Autodesk Fusion 360 part; units mm, degrees
(part 13 of 40)
  line L5726 (150.1623, 135.5673) -> (150.0253, 135.4891) construction
  line L5727 (150.0253, 135.4891) -> (149.8888, 135.4096) construction
  line L5728 (149.8888, 135.4096) -> (149.7528, 135.3289) construction
  line L5729 (149.7528, 135.3289) -> (149.6172, 135.247) construction
  line L5730 (149.6172, 135.247) -> (149.4822, 135.1637) construction
  line L5731 (149.4822, 135.1637) -> (149.3477, 135.0792) construction
  line L5732 (149.3477, 135.0792) -> (149.2136, 134.9936) construction
  line L5733 (149.2136, 134.9936) -> (149.08, 134.9068) construction
  line L5734 (149.08, 134.9068) -> (148.9468, 134.819) construction
  line L5735 (148.9468, 134.819) -> (148.814, 134.7302) construction
  line L5736 (148.814, 134.7302) -> (148.6817, 134.6403) construction
  line L5737 (148.6817, 134.6403) -> (148.5499, 134.5494) construction
  line L5738 (148.5499, 134.5494) -> (148.4185, 134.4575) construction
  line L5739 (148.4185, 134.4575) -> (148.2875, 134.3646) construction
  line L5740 (148.2875, 134.3646) -> (148.157, 134.2707) construction
  line L5741 (148.157, 134.2707) -> (148.027, 134.1758) construction
  line L5742 (148.027, 134.1758) -> (147.8974, 134.08) construction
  line L5743 (147.8974, 134.08) -> (147.7682, 133.9832) construction
  line L5744 (147.7682, 133.9832) -> (147.6394, 133.8854) construction
  line L5745 (147.6394, 133.8854) -> (147.5111, 133.7868) construction
  line L5746 (147.5111, 133.7868) -> (147.3832, 133.6873) construction
  line L5747 (147.3832, 133.6873) -> (147.2558, 133.5869) construction
  line L5748 (147.2558, 133.5869) -> (147.1288, 133.4856) construction
  line L5749 (147.1288, 133.4856) -> (147.0022, 133.3834) construction
  line L5750 (147.0022, 133.3834) -> (146.876, 133.2804) construction
  line L5751 (146.876, 133.2804) -> (146.7503, 133.1765) construction
  line L5752 (146.7503, 133.1765) -> (146.625, 133.0717) construction
  line L5753 (146.625, 133.0717) -> (146.5002, 132.9662) construction
  line L5754 (146.5002, 132.9662) -> (146.3758, 132.8598) construction
  line L5755 (146.3758, 132.8598) -> (146.2518, 132.7526) construction
  line L5756 (146.2518, 132.7526) -> (146.1282, 132.6445) construction
  line L5757 (146.1282, 132.6445) -> (146.0051, 132.5357) construction
  line L5758 (146.0051, 132.5357) -> (145.8823, 132.4261) construction
  line L5759 (145.8823, 132.4261) -> (145.7601, 132.3158) construction
  line L5760 (145.7601, 132.3158) -> (145.6382, 132.2046) construction
  line L5761 (145.6382, 132.2046) -> (145.5168, 132.0927) construction
  line L5762 (145.5168, 132.0927) -> (145.3958, 131.98) construction
  line L5763 (145.3958, 131.98) -> (145.2752, 131.8665) construction
  line L5764 (145.2752, 131.8665) -> (145.1551, 131.7523) construction
  line L5765 (145.1551, 131.7523) -> (145.0354, 131.6374) construction
  line L5766 (145.0354, 131.6374) -> (144.9161, 131.5218) construction
  line L5767 (144.9161, 131.5218) -> (144.7973, 131.4054) construction
  line L5768 (144.7973, 131.4054) -> (144.6789, 131.2882) construction
  line L5769 (144.6789, 131.2882) -> (144.5609, 131.1704) construction
  line L5770 (144.5609, 131.1704) -> (144.4433, 131.0519) construction
  line L5771 (144.4433, 131.0519) -> (144.3262, 130.9326) construction
  line L5772 (144.3262, 130.9326) -> (144.2095, 130.8127) construction
  line L5773 (144.2095, 130.8127) -> (144.0932, 130.6921) construction
  line L5774 (144.0932, 130.6921) -> (143.9774, 130.5707) construction
  line L5775 (143.9774, 130.5707) -> (143.862, 130.4488) construction
  line L5776 (143.862, 130.4488) -> (143.747, 130.3261) construction
  line L5777 (143.747, 130.3261) -> (143.6553, 130.2274) construction
  line L5778 (143.6553, 130.2274) -> (143.5868, 130.1531) construction
  line L5779 (143.5868, 130.1531) -> (143.5412, 130.1034) construction
  line L5780 (143.5412, 130.1034) -> (143.5184, 130.0785) construction
  arc A153 (161.0254, 119.7202) -> (161.7599, 122.4018) centre (160.0059, 121.4408) ccw
  arc A154 (152.9878, 155.5428) -> (155.1583, 157.2806) centre (153.1745, 157.5341) ccw
  arc A155 (143.5184, 130.0785) -> (144.9129, 125.7868) centre (212.132, 150) ccw
  arc A156 (160.1966, 125.4699) -> (161.7599, 122.4018) centre (212.132, 150) ccw
  line L5781 (152.9878, 155.5428) -> (151.3635, 155.6951)
  arc A157 (154.1697, 136.995) -> (155.697, 139.3184) centre (153.7319, 138.9465) ccw
  arc A158 (155.1583, 142.7194) -> (155.697, 139.3184) centre (212.132, 150) ccw
  spline S77 degree 5 poles (151.3635, 144.3049) (151.3327, 144.3021) (151.2711, 144.2971) (151.1787, 144.2922) (151.0554, 144.2903) (150.901, 144.2944) (150.7464, 144.3031) (150.5917, 144.3146) (150.437, 144.3277) (150.2822, 144.3417) (150.1275, 144.3569) (149.9727, 144.3735) (149.818, 144.392) (149.6632, 144.4129) (149.5085, 144.4359) (149.3538, 144.461) (149.1991, 144.4879) (149.0445, 144.5162) (148.8899, 144.5458) (148.7354, 144.5767) (148.5809, 144.6087) (148.4265, 144.6421) (148.2722, 144.6768) (148.118, 144.7129) (147.9638, 144.7503) (147.8098, 144.7891) (147.6558, 144.8291) (147.5019, 144.8703) (147.3481, 144.9127) (147.1944, 144.9561) (147.0408, 145.0007) (146.8873, 145.0464) (146.734, 145.0932) (146.5807, 145.1411) (146.4276, 145.1901) (146.2746, 145.2401) (146.1217, 145.2913) (145.9689, 145.3434) (145.8162, 145.3965) (145.6637, 145.4507) (145.5114, 145.5058) (145.3591, 145.562) (145.207, 145.619) (145.055, 145.6771) (144.9032, 145.7361) (144.7516, 145.7961) (144.6, 145.857) (144.4487, 145.9188) (144.2975, 145.9815) (144.1464, 146.0452) (143.9955, 146.1097) (143.8448, 146.1751) (143.6942, 146.2415) (143.5438, 146.3087) (143.3936, 146.3767) (143.2435, 146.4457) (143.0936, 146.5154) (142.9439, 146.5861) (142.7944, 146.6575) (142.645, 146.7299) (142.4958, 146.803) (142.3468, 146.877) (142.198, 146.9518) (142.0494, 147.0274) (141.9009, 147.1038) (141.7527, 147.181) (141.6046, 147.259) (141.4568, 147.3378) (141.3091, 147.4174) (141.1617, 147.4977) (141.0144, 147.5789) (140.8968, 147.6444) (140.8086, 147.6939) (140.7499, 147.7271) (140.7205, 147.7437) knots 0 0 0 0 0 0 0.01428571 0.02857143 0.04285714 0.05714286 0.07142857 0.08571429 0.1 0.11428571 0.12857143 0.14285714 0.15714286 0.17142857 0.18571429 0.2 0.21428571 0.22857143 0.24285714 0.25714286 0.27142857 0.28571429 0.3 0.31428571 0.32857143 0.34285714 0.35714286 0.37142857 0.38571429 0.4 0.41428571 0.42857143 0.44285714 0.45714286 0.47142857 0.48571429 0.5 0.51428571 0.52857143 0.54285714 0.55714286 0.57142857 0.58571429 0.6 0.61428571 0.62857143 0.64285714 0.65714286 0.67142857 0.68571429 0.7 0.71428571 0.72857143 0.74285714 0.75714286 0.77142857 0.78571429 0.8 0.81428571 0.82857143 0.84285714 0.85714286 0.87142857 0.88571429 0.9 0.91428571 0.92857143 0.94285714 0.95714286 0.97142857 0.98571429 1 1 1 1 1 1
  line L5782 (151.3635, 144.3049) -> (151.3327, 144.3021) construction
  line L5783 (151.3327, 144.3021) -> (151.2711, 144.2971) construction
  line L5784 (151.2711, 144.2971) -> (151.1787, 144.2922) construction
  line L5785 (151.1787, 144.2922) -> (151.0554, 144.2903) construction
  line L5786 (151.0554, 144.2903) -> (150.901, 144.2944) construction
  line L5787 (150.901, 144.2944) -> (150.7464, 144.3031) construction
  line L5788 (150.7464, 144.3031) -> (150.5917, 144.3146) construction
  line L5789 (150.5917, 144.3146) -> (150.437, 144.3277) construction
  line L5790 (150.437, 144.3277) -> (150.2822, 144.3417) construction
  line L5791 (150.2822, 144.3417) -> (150.1275, 144.3569) construction
  line L5792 (150.1275, 144.3569) -> (149.9727, 144.3735) construction
  line L5793 (149.9727, 144.3735) -> (149.818, 144.392) construction
  line L5794 (149.818, 144.392) -> (149.6632, 144.4129) construction
  line L5795 (149.6632, 144.4129) -> (149.5085, 144.4359) construction
  line L5796 (149.5085, 144.4359) -> (149.3538, 144.461) construction
  line L5797 (149.3538, 144.461) -> (149.1991, 144.4879) construction
  line L5798 (149.1991, 144.4879) -> (149.0445, 144.5162) construction
  line L5799 (149.0445, 144.5162) -> (148.8899, 144.5458) construction
  line L5800 (148.8899, 144.5458) -> (148.7354, 144.5767) construction
  line L5801 (148.7354, 144.5767) -> (148.5809, 144.6087) construction
  line L5802 (148.5809, 144.6087) -> (148.4265, 144.6421) construction
  line L5803 (148.4265, 144.6421) -> (148.2722, 144.6768) construction
  line L5804 (148.2722, 144.6768) -> (148.118, 144.7129) construction
  line L5805 (148.118, 144.7129) -> (147.9638, 144.7503) construction
  line L5806 (147.9638, 144.7503) -> (147.8098, 144.7891) construction
  line L5807 (147.8098, 144.7891) -> (147.6558, 144.8291) construction
  line L5808 (147.6558, 144.8291) -> (147.5019, 144.8703) construction
  line L5809 (147.5019, 144.8703) -> (147.3481, 144.9127) construction
  line L5810 (147.3481, 144.9127) -> (147.1944, 144.9561) construction
  line L5811 (147.1944, 144.9561) -> (147.0408, 145.0007) construction
  line L5812 (147.0408, 145.0007) -> (146.8873, 145.0464) construction
  line L5813 (146.8873, 145.0464) -> (146.734, 145.0932) construction
  line L5814 (146.734, 145.0932) -> (146.5807, 145.1411) construction
  line L5815 (146.5807, 145.1411) -> (146.4276, 145.1901) construction
  line L5816 (146.4276, 145.1901) -> (146.2746, 145.2401) construction
  line L5817 (146.2746, 145.2401) -> (146.1217, 145.2913) construction
  line L5818 (146.1217, 145.2913) -> (145.9689, 145.3434) construction
  line L5819 (145.9689, 145.3434) -> (145.8162, 145.3965) construction
  line L5820 (145.8162, 145.3965) -> (145.6637, 145.4507) construction
  line L5821 (145.6637, 145.4507) -> (145.5114, 145.5058) construction
  line L5822 (145.5114, 145.5058) -> (145.3591, 145.562) construction
  line L5823 (145.3591, 145.562) -> (145.207, 145.619) construction
  line L5824 (145.207, 145.619) -> (145.055, 145.6771) construction
  line L5825 (145.055, 145.6771) -> (144.9032, 145.7361) construction
  line L5826 (144.9032, 145.7361) -> (144.7516, 145.7961) construction
  line L5827 (144.7516, 145.7961) -> (144.6, 145.857) construction
  line L5828 (144.6, 145.857) -> (144.4487, 145.9188) construction
  line L5829 (144.4487, 145.9188) -> (144.2975, 145.9815) construction
  line L5830 (144.2975, 145.9815) -> (144.1464, 146.0452) construction
  line L5831 (144.1464, 146.0452) -> (143.9955, 146.1097) construction
  line L5832 (143.9955, 146.1097) -> (143.8448, 146.1751) construction
  line L5833 (143.8448, 146.1751) -> (143.6942, 146.2415) construction
  line L5834 (143.6942, 146.2415) -> (143.5438, 146.3087) construction
  line L5835 (143.5438, 146.3087) -> (143.3936, 146.3767) construction
  line L5836 (143.3936, 146.3767) -> (143.2435, 146.4457) construction
  line L5837 (143.2435, 146.4457) -> (143.0936, 146.5154) construction
  line L5838 (143.0936, 146.5154) -> (142.9439, 146.5861) construction
  line L5839 (142.9439, 146.5861) -> (142.7944, 146.6575) construction
  line L5840 (142.7944, 146.6575) -> (142.645, 146.7299) construction
  line L5841 (142.645, 146.7299) -> (142.4958, 146.803) construction
  line L5842 (142.4958, 146.803) -> (142.3468, 146.877) construction
  line L5843 (142.3468, 146.877) -> (142.198, 146.9518) construction
  line L5844 (142.198, 146.9518) -> (142.0494, 147.0274) construction
  line L5845 (142.0494, 147.0274) -> (141.9009, 147.1038) construction
  line L5846 (141.9009, 147.1038) -> (141.7527, 147.181) construction
  line L5847 (141.7527, 147.181) -> (141.6046, 147.259) construction
  line L5848 (141.6046, 147.259) -> (141.4568, 147.3378) construction
  line L5849 (141.4568, 147.3378) -> (141.3091, 147.4174) construction
  line L5850 (141.3091, 147.4174) -> (141.1617, 147.4977) construction
  line L5851 (141.1617, 147.4977) -> (141.0144, 147.5789) construction
  line L5852 (141.0144, 147.5789) -> (140.8968, 147.6444) construction
  line L5853 (140.8968, 147.6444) -> (140.8086, 147.6939) construction
  line L5854 (140.8086, 147.6939) -> (140.7499, 147.7271) construction
  line L5855 (140.7499, 147.7271) -> (140.7205, 147.7437) construction
  arc A159 (155.697, 160.6816) -> (154.1697, 163.005) centre (153.7319, 161.0535) ccw
  arc A160 (154.1697, 136.995) -> (155.697, 139.3184) centre (153.7319, 138.9465) ccw
  arc A161 (255.932, 206.4469) -> (252.2812, 209.0993) centre (212.132, 150) ccw
  spline S78 degree 5 poles (152.5778, 163.3622) (152.5477, 163.369) (152.4876, 163.3833) (152.3982, 163.4071) (152.2803, 163.4435) (152.1347, 163.4951) (151.9904, 163.5511) (151.8468, 163.6099) (151.7037, 163.6701) (151.5609, 163.7313) (151.4184, 163.7935) (151.2763, 163.8571) (151.1349, 163.9226) (150.9941, 163.9902) (150.8541, 164.06) (150.7147, 164.1316) (150.5759, 164.205) (150.4376, 164.2797) (150.2998, 164.3557) (150.1623, 164.4327) (150.0253, 164.5109) (149.8888, 164.5904) (149.7528, 164.6711) (149.6172, 164.753) (149.4822, 164.8363) (149.3477, 164.9208) (149.2136, 165.0064) (149.08, 165.0932) (148.9468, 165.181) (148.814, 165.2698) (148.6817, 165.3597) (148.5499, 165.4506) (148.4185, 165.5425) (148.2875, 165.6354) (148.157, 165.7293) (148.027, 165.8242) (147.8974, 165.92) (147.7682, 166.0168) (147.6394, 166.1146) (147.5111, 166.2132) (147.3832, 166.3127) (147.2558, 166.4131) (147.1288, 166.5144) (147.0022, 166.6166) (146.876, 166.7196) (146.7503, 166.8235) (146.625, 166.9283) (146.5002, 167.0338) (146.3758, 167.1402) (146.2518, 167.2474) (146.1282, 167.3555) (146.0051, 167.4643) (145.8823, 167.5739) (145.7601, 167.6842) (145.6382, 167.7954) (145.5168, 167.9073) (145.3958, 168.02) (145.2752, 168.1335) (145.1551, 168.2477) (145.0354, 168.3626) (144.9161, 168.4782) (144.7973, 168.5946) (144.6789, 168.7118) (144.5609, 168.8296) (144.4433, 168.9481) (144.3262, 169.0674) (144.2095, 169.1873) (144.0932, 169.3079) (143.9774, 169.4293) (143.862, 169.5512) (143.747, 169.6739) (143.6553, 169.7726) (143.5868, 169.8469) (143.5412, 169.8966) (143.5184, 169.9215) knots 0 0 0 0 0 0 0.01428571 0.02857143 0.04285714 0.05714286 0.07142857 0.08571429 0.1 0.11428571 0.12857143 0.14285714 0.15714286 0.17142857 0.18571429 0.2 0.21428571 0.22857143 0.24285714 0.25714286 0.27142857 0.28571429 0.3 0.31428571 0.32857143 0.34285714 0.35714286 0.37142857 0.38571429 0.4 0.41428571 0.42857143 0.44285714 0.45714286 0.47142857 0.48571429 0.5 0.51428571 0.52857143 0.54285714 0.55714286 0.57142857 0.58571429 0.6 0.61428571 0.62857143 0.64285714 0.65714286 0.67142857 0.68571429 0.7 0.71428571 0.72857143 0.74285714 0.75714286 0.77142857 0.78571429 0.8 0.81428571 0.82857143 0.84285714 0.85714286 0.87142857 0.88571429 0.9 0.91428571 0.92857143 0.94285714 0.95714286 0.97142857 0.98571429 1 1 1 1 1 1
  line L5856 (152.5778, 163.3622) -> (152.5477, 163.369) construction
  line L5857 (152.5477, 163.369) -> (152.4876, 163.3833) construction
  line L5858 (152.4876, 163.3833) -> (152.3982, 163.4071) construction
  line L5859 (152.3982, 163.4071) -> (152.2803, 163.4435) construction
  line L5860 (152.2803, 163.4435) -> (152.1347, 163.4951) construction
  line L5861 (152.1347, 163.4951) -> (151.9904, 163.5511) construction
  line L5862 (151.9904, 163.5511) -> (151.8468, 163.6099) construction
  line L5863 (151.8468, 163.6099) -> (151.7037, 163.6701) construction
  line L5864 (151.7037, 163.6701) -> (151.5609, 163.7313) construction
  line L5865 (151.5609, 163.7313) -> (151.4184, 163.7935) construction
  line L5866 (151.4184, 163.7935) -> (151.2763, 163.8571) construction
  line L5867 (151.2763, 163.8571) -> (151.1349, 163.9226) construction
  line L5868 (151.1349, 163.9226) -> (150.9941, 163.9902) construction
  line L5869 (150.9941, 163.9902) -> (150.8541, 164.06) construction
  line L5870 (150.8541, 164.06) -> (150.7147, 164.1316) construction
  line L5871 (150.7147, 164.1316) -> (150.5759, 164.205) construction
  line L5872 (150.5759, 164.205) -> (150.4376, 164.2797) construction
  line L5873 (150.4376, 164.2797) -> (150.2998, 164.3557) construction
  line L5874 (150.2998, 164.3557) -> (150.1623, 164.4327) construction
  line L5875 (150.1623, 164.4327) -> (150.0253, 164.5109) construction
  line L5876 (150.0253, 164.5109) -> (149.8888, 164.5904) construction
  line L5877 (149.8888, 164.5904) -> (149.7528, 164.6711) construction
  line L5878 (149.7528, 164.6711) -> (149.6172, 164.753) construction
  line L5879 (149.6172, 164.753) -> (149.4822, 164.8363) construction
  line L5880 (149.4822, 164.8363) -> (149.3477, 164.9208) construction
  line L5881 (149.3477, 164.9208) -> (149.2136, 165.0064) construction
  line L5882 (149.2136, 165.0064) -> (149.08, 165.0932) construction
  line L5883 (149.08, 165.0932) -> (148.9468, 165.181) construction
  line L5884 (148.9468, 165.181) -> (148.814, 165.2698) construction
  line L5885 (148.814, 165.2698) -> (148.6817, 165.3597) construction
  line L5886 (148.6817, 165.3597) -> (148.5499, 165.4506) construction
  line L5887 (148.5499, 165.4506) -> (148.4185, 165.5425) construction
  line L5888 (148.4185, 165.5425) -> (148.2875, 165.6354) construction
  line L5889 (148.2875, 165.6354) -> (148.157, 165.7293) construction
  line L5890 (148.157, 165.7293) -> (148.027, 165.8242) construction
  line L5891 (148.027, 165.8242) -> (147.8974, 165.92) construction
  line L5892 (147.8974, 165.92) -> (147.7682, 166.0168) construction
  line L5893 (147.7682, 166.0168) -> (147.6394, 166.1146) construction
  line L5894 (147.6394, 166.1146) -> (147.5111, 166.2132) construction
  line L5895 (147.5111, 166.2132) -> (147.3832, 166.3127) construction
  line L5896 (147.3832, 166.3127) -> (147.2558, 166.4131) construction
  line L5897 (147.2558, 166.4131) -> (147.1288, 166.5144) construction
  line L5898 (147.1288, 166.5144) -> (147.0022, 166.6166) construction
  line L5899 (147.0022, 166.6166) -> (146.876, 166.7196) construction
  line L5900 (146.876, 166.7196) -> (146.7503, 166.8235) construction
  line L5901 (146.7503, 166.8235) -> (146.625, 166.9283) construction
  line L5902 (146.625, 166.9283) -> (146.5002, 167.0338) construction
  line L5903 (146.5002, 167.0338) -> (146.3758, 167.1402) construction
  line L5904 (146.3758, 167.1402) -> (146.2518, 167.2474) construction
  line L5905 (146.2518, 167.2474) -> (146.1282, 167.3555) construction
  line L5906 (146.1282, 167.3555) -> (146.0051, 167.4643) construction
  line L5907 (146.0051, 167.4643) -> (145.8823, 167.5739) construction
  line L5908 (145.8823, 167.5739) -> (145.7601, 167.6842) construction
  line L5909 (145.7601, 167.6842) -> (145.6382, 167.7954) construction
  line L5910 (145.6382, 167.7954) -> (145.5168, 167.9073) construction
  line L5911 (145.5168, 167.9073) -> (145.3958, 168.02) construction
  line L5912 (145.3958, 168.02) -> (145.2752, 168.1335) construction
  line L5913 (145.2752, 168.1335) -> (145.1551, 168.2477) construction
  line L5914 (145.1551, 168.2477) -> (145.0354, 168.3626) construction
  line L5915 (145.0354, 168.3626) -> (144.9161, 168.4782) construction
  line L5916 (144.9161, 168.4782) -> (144.7973, 168.5946) construction
  line L5917 (144.7973, 168.5946) -> (144.6789, 168.7118) construction
  line L5918 (144.6789, 168.7118) -> (144.5609, 168.8296) construction
  line L5919 (144.5609, 168.8296) -> (144.4433, 168.9481) construction
  line L5920 (144.4433, 168.9481) -> (144.3262, 169.0674) construction
  line L5921 (144.3262, 169.0674) -> (144.2095, 169.1873) construction
  line L5922 (144.2095, 169.1873) -> (144.0932, 169.3079) construction
  line L5923 (144.0932, 169.3079) -> (143.9774, 169.4293) construction
  line L5924 (143.9774, 169.4293) -> (143.862, 169.5512) construction
  line L5925 (143.862, 169.5512) -> (143.747, 169.6739) construction
  line L5926 (143.747, 169.6739) -> (143.6553, 169.7726) construction
  line L5927 (143.6553, 169.7726) -> (143.5868, 169.8469) construction
  line L5928 (143.5868, 169.8469) -> (143.5412, 169.8966) construction
  line L5929 (143.5412, 169.8966) -> (143.5184, 169.9215) construction
  spline S79 degree 5 poles (156.0975, 174.1948) (156.0692, 174.2071) (156.0122, 174.2308) (155.9258, 174.264) (155.8091, 174.3039) (155.6609, 174.3478) (155.5112, 174.3873) (155.3606, 174.4241) (155.2094, 174.4595) (155.0579, 174.494) (154.906, 174.5274) (154.7537, 174.5594) (154.6008, 174.5896) (154.4472, 174.6176) (154.2929, 174.6435) (154.138, 174.6674) (153.9826, 174.6897) (153.8268, 174.7105) (153.6706, 174.7301) (153.5141, 174.7485) (153.3573, 174.7658) (153.2002, 174.7818) (153.0427, 174.7965) (152.8849, 174.8098) (152.7267, 174.8218) (152.5682, 174.8325) (152.4094, 174.842) (152.2503, 174.8504) (152.0909, 174.8577) (151.9313, 174.8638) (151.7715, 174.8689) (151.6114, 174.8729) (151.4511, 174.8757) (151.2905, 174.8776) (151.1297, 174.8783) (150.9687, 174.878) (150.8075, 174.8766) (150.6461, 174.8742) (150.4845, 174.8708) (150.3227, 174.8665) (150.1608, 174.8611) (149.9986, 174.8548) (149.8363, 174.8475) (149.6739, 174.8392) (149.5113, 174.83) (149.3485, 174.8199) (149.1856, 174.8088) (149.0225, 174.7967) (148.8593, 174.7838) (148.696, 174.77) (148.5325, 174.7552) (148.3689, 174.7396) (148.2052, 174.723) (148.0414, 174.7056) (147.8775, 174.6873) (147.7135, 174.6681) (147.5494, 174.648) (147.3852, 174.6271) (147.2209, 174.6054) (147.0565, 174.5828) (146.892, 174.5593) (146.7274, 174.535) (146.5628, 174.5098) (146.398, 174.4839) (146.2333, 174.4571) (146.0684, 174.4294) (145.9035, 174.401) (145.7385, 174.3718) (145.5735, 174.3417) (145.4084, 174.3108) (145.2433, 174.2792) (145.1112, 174.2532) (145.0121, 174.2334) (144.946, 174.22) (144.9129, 174.2132) knots 0 0 0 0 0 0 0.01428571 0.02857143 0.04285714 0.05714286 0.07142857 0.08571429 0.1 0.11428571 0.12857143 0.14285714 0.15714286 0.17142857 0.18571429 0.2 0.21428571 0.22857143 0.24285714 0.25714286 0.27142857 0.28571429 0.3 0.31428571 0.32857143 0.34285714 0.35714286 0.37142857 0.38571429 0.4 0.41428571 0.42857143 0.44285714 0.45714286 0.47142857 0.48571429 0.5 0.51428571 0.52857143 0.54285714 0.55714286 0.57142857 0.58571429 0.6 0.61428571 0.62857143 0.64285714 0.65714286 0.67142857 0.68571429 0.7 0.71428571 0.72857143 0.74285714 0.75714286 0.77142857 0.78571429 0.8 0.81428571 0.82857143 0.84285714 0.85714286 0.87142857 0.88571429 0.9 0.91428571 0.92857143 0.94285714 0.95714286 0.97142857 0.98571429 1 1 1 1 1 1
  line L5930 (156.0975, 174.1948) -> (156.0692, 174.2071) construction
  line L5931 (156.0692, 174.2071) -> (156.0122, 174.2308) construction
  line L5932 (156.0122, 174.2308) -> (155.9258, 174.264) construction
  line L5933 (155.9258, 174.264) -> (155.8091, 174.3039) construction
  line L5934 (155.8091, 174.3039) -> (155.6609, 174.3478) construction
  line L5935 (155.6609, 174.3478) -> (155.5112, 174.3873) construction
  line L5936 (155.5112, 174.3873) -> (155.3606, 174.4241) construction
  line L5937 (155.3606, 174.4241) -> (155.2094, 174.4595) construction
  line L5938 (155.2094, 174.4595) -> (155.0579, 174.494) construction
  line L5939 (155.0579, 174.494) -> (154.906, 174.5274) construction
  line L5940 (154.906, 174.5274) -> (154.7537, 174.5594) construction
  line L5941 (154.7537, 174.5594) -> (154.6008, 174.5896) construction
  line L5942 (154.6008, 174.5896) -> (154.4472, 174.6176) construction
  line L5943 (154.4472, 174.6176) -> (154.2929, 174.6435) construction
  line L5944 (154.2929, 174.6435) -> (154.138, 174.6674) construction
  line L5945 (154.138, 174.6674) -> (153.9826, 174.6897) construction
  line L5946 (153.9826, 174.6897) -> (153.8268, 174.7105) construction
  line L5947 (153.8268, 174.7105) -> (153.6706, 174.7301) construction
  line L5948 (153.6706, 174.7301) -> (153.5141, 174.7485) construction
  line L5949 (153.5141, 174.7485) -> (153.3573, 174.7658) construction
  line L5950 (153.3573, 174.7658) -> (153.2002, 174.7818) construction
  line L5951 (153.2002, 174.7818) -> (153.0427, 174.7965) construction
  line L5952 (153.0427, 174.7965) -> (152.8849, 174.8098) construction
  line L5953 (152.8849, 174.8098) -> (152.7267, 174.8218) construction
  line L5954 (152.7267, 174.8218) -> (152.5682, 174.8325) construction
  line L5955 (152.5682, 174.8325) -> (152.4094, 174.842) construction
  line L5956 (152.4094, 174.842) -> (152.2503, 174.8504) construction
  line L5957 (152.2503, 174.8504) -> (152.0909, 174.8577) construction
  line L5958 (152.0909, 174.8577) -> (151.9313, 174.8638) construction
  line L5959 (151.9313, 174.8638) -> (151.7715, 174.8689) construction
  line L5960 (151.7715, 174.8689) -> (151.6114, 174.8729) construction
  line L5961 (151.6114, 174.8729) -> (151.4511, 174.8757) construction
  line L5962 (151.4511, 174.8757) -> (151.2905, 174.8776) construction
  line L5963 (151.2905, 174.8776) -> (151.1297, 174.8783) construction
  line L5964 (151.1297, 174.8783) -> (150.9687, 174.878) construction
  line L5965 (150.9687, 174.878) -> (150.8075, 174.8766) construction
  line L5966 (150.8075, 174.8766) -> (150.6461, 174.8742) construction
  line L5967 (150.6461, 174.8742) -> (150.4845, 174.8708) construction
  line L5968 (150.4845, 174.8708) -> (150.3227, 174.8665) construction
  line L5969 (150.3227, 174.8665) -> (150.1608, 174.8611) construction
  line L5970 (150.1608, 174.8611) -> (149.9986, 174.8548) construction
  line L5971 (149.9986, 174.8548) -> (149.8363, 174.8475) construction
  line L5972 (149.8363, 174.8475) -> (149.6739, 174.8392) construction
  line L5973 (149.6739, 174.8392) -> (149.5113, 174.83) construction
  line L5974 (149.5113, 174.83) -> (149.3485, 174.8199) construction
  line L5975 (149.3485, 174.8199) -> (149.1856, 174.8088) construction
  line L5976 (149.1856, 174.8088) -> (149.0225, 174.7967) construction
  line L5977 (149.0225, 174.7967) -> (148.8593, 174.7838) construction
  line L5978 (148.8593, 174.7838) -> (148.696, 174.77) construction
  line L5979 (148.696, 174.77) -> (148.5325, 174.7552) construction
  line L5980 (148.5325, 174.7552) -> (148.3689, 174.7396) construction
  line L5981 (148.3689, 174.7396) -> (148.2052, 174.723) construction
  line L5982 (148.2052, 174.723) -> (148.0414, 174.7056) construction
  line L5983 (148.0414, 174.7056) -> (147.8775, 174.6873) construction
  line L5984 (147.8775, 174.6873) -> (147.7135, 174.6681) construction
  line L5985 (147.7135, 174.6681) -> (147.5494, 174.648) construction
  line L5986 (147.5494, 174.648) -> (147.3852, 174.6271) construction
  line L5987 (147.3852, 174.6271) -> (147.2209, 174.6054) construction
  line L5988 (147.2209, 174.6054) -> (147.0565, 174.5828) construction
  line L5989 (147.0565, 174.5828) -> (146.892, 174.5593) construction
  line L5990 (146.892, 174.5593) -> (146.7274, 174.535) construction
  line L5991 (146.7274, 174.535) -> (146.5628, 174.5098) construction
  line L5992 (146.5628, 174.5098) -> (146.398, 174.4839) construction
  line L5993 (146.398, 174.4839) -> (146.2333, 174.4571) construction
  line L5994 (146.2333, 174.4571) -> (146.0684, 174.4294) construction
  line L5995 (146.0684, 174.4294) -> (145.9035, 174.401) construction
  line L5996 (145.9035, 174.401) -> (145.7385, 174.3718) construction
  line L5997 (145.7385, 174.3718) -> (145.5735, 174.3417) construction
  line L5998 (145.5735, 174.3417) -> (145.4084, 174.3108) construction
  line L5999 (145.4084, 174.3108) -> (145.2433, 174.2792) construction
  line L6000 (145.2433, 174.2792) -> (145.1112, 174.2532) construction
  line L6001 (145.1112, 174.2532) -> (145.0121, 174.2334) construction
  line L6002 (145.0121, 174.2334) -> (144.946, 174.22) construction
  line L6003 (144.946, 174.22) -> (144.9129, 174.2132) construction
  dimension "d60" = 50
  constraint coincident L0.end L1.start
  constraint perpendicular L1 L3
  measures "d60" distance of L0.end L3.end
sketch "Base Circle" plane through (0, 0, 0) normal (0, 0, 1) x (1, 0, 0)
  circle A0 centre (0, 0) radius 57.437
  circle A1 centre (0, 0) radius 2.3
extrude "Extrude4" add sketch "Base Circle" along normal blind 4.2 separate body makes body 6
sketch "Gear Tooth" plane through (0, 0, 0) normal (0, 0, 1) x (1, 0, 0)
  spline S0 degree 5 poles (60.7685, -5.6951) (60.7993, -5.6979) (60.8609, -5.7029) (60.9533, -5.7078) (61.0766, -5.7097) (61.231, -5.7056) (61.3856, -5.6969) (61.5403, -5.6854) (61.695, -5.6723) (61.8498, -5.6583) (62.0045, -5.6431) (62.1593, -5.6265) (62.314, -5.608) (62.4688, -5.5871) (62.6235, -5.5641) (62.7782, -5.539) (62.9329, -5.5121) (63.0875, -5.4838) (63.2421, -5.4542) (63.3966, -5.4233) (63.5511, -5.3913) (63.7055, -5.3579) (63.8598, -5.3232) (64.014, -5.2871) (64.1682, -5.2497) (64.3222, -5.2109) (64.4762, -5.1709) (64.6301, -5.1297) (64.7839, -5.0873) (64.9376, -5.0439) (65.0912, -4.9993) (65.2447, -4.9536) (65.398, -4.9068) (65.5513, -4.8589) (65.7044, -4.8099) (65.8574, -4.7599) (66.0103, -4.7087) (66.1631, -4.6566) (66.3158, -4.6035) (66.4683, -4.5493) (66.6206, -4.4942) (66.7729, -4.438) (66.925, -4.381) (67.077, -4.3229) (67.2288, -4.2639) (67.3804, -4.2039) (67.532, -4.143) (67.6833, -4.0812) (67.8345, -4.0185) (67.9856, -3.9548) (68.1365, -3.8903) (68.2872, -3.8249) (68.4378, -3.7585) (68.5882, -3.6913) (68.7384, -3.6233) (68.8885, -3.5543) (69.0384, -3.4846) (69.1881, -3.4139) (69.3376, -3.3425) (69.487, -3.2701) (69.6362, -3.197) (69.7852, -3.123) (69.934, -3.0482) (70.0826, -2.9726) (70.2311, -2.8962) (70.3793, -2.819) (70.5274, -2.741) (70.6752, -2.6622) (70.8229, -2.5826) (70.9703, -2.5023) (71.1176, -2.4211) (71.2352, -2.3556) (71.3234, -2.3061) (71.3821, -2.2729) (71.4115, -2.2563) knots 0 0 0 0 0 0 0.01428571 0.02857143 0.04285714 0.05714286 0.07142857 0.08571429 0.1 0.11428571 0.12857143 0.14285714 0.15714286 0.17142857 0.18571429 0.2 0.21428571 0.22857143 0.24285714 0.25714286 0.27142857 0.28571429 0.3 0.31428571 0.32857143 0.34285714 0.35714286 0.37142857 0.38571429 0.4 0.41428571 0.42857143 0.44285714 0.45714286 0.47142857 0.48571429 0.5 0.51428571 0.52857143 0.54285714 0.55714286 0.57142857 0.58571429 0.6 0.61428571 0.62857143 0.64285714 0.65714286 0.67142857 0.68571429 0.7 0.71428571 0.72857143 0.74285714 0.75714286 0.77142857 0.78571429 0.8 0.81428571 0.82857143 0.84285714 0.85714286 0.87142857 0.88571429 0.9 0.91428571 0.92857143 0.94285714 0.95714286 0.97142857 0.98571429 1 1 1 1 1 1
  spline S1 degree 5 poles (60.7685, 5.6951) (60.7993, 5.6979) (60.8609, 5.7029) (60.9533, 5.7078) (61.0766, 5.7097) (61.231, 5.7056) (61.3856, 5.6969) (61.5403, 5.6854) (61.695, 5.6723) (61.8498, 5.6583) (62.0045, 5.6431) (62.1593, 5.6265) (62.314, 5.608) (62.4688, 5.5871) (62.6235, 5.5641) (62.7782, 5.539) (62.9329, 5.5121) (63.0875, 5.4838) (63.2421, 5.4542) (63.3966, 5.4233) (63.5511, 5.3913) (63.7055, 5.3579) (63.8598, 5.3232) (64.014, 5.2871) (64.1682, 5.2497) (64.3222, 5.2109) (64.4762, 5.1709) (64.6301, 5.1297) (64.7839, 5.0873) (64.9376, 5.0439) (65.0912, 4.9993) (65.2447, 4.9536) (65.398, 4.9068) (65.5513, 4.8589) (65.7044, 4.8099) (65.8574, 4.7599) (66.0103, 4.7087) (66.1631, 4.6566) (66.3158, 4.6035) (66.4683, 4.5493) (66.6206, 4.4942) (66.7729, 4.438) (66.925, 4.381) (67.077, 4.3229) (67.2288, 4.2639) (67.3804, 4.2039) (67.532, 4.143) (67.6833, 4.0812) (67.8345, 4.0185) (67.9856, 3.9548) (68.1365, 3.8903) (68.2872, 3.8249) (68.4378, 3.7585) (68.5882, 3.6913) (68.7384, 3.6233) (68.8885, 3.5543) (69.0384, 3.4846) (69.1881, 3.4139) (69.3376, 3.3425) (69.487, 3.2701) (69.6362, 3.197) (69.7852, 3.123) (69.934, 3.0482) (70.0826, 2.9726) (70.2311, 2.8962) (70.3793, 2.819) (70.5274, 2.741) (70.6752, 2.6622) (70.8229, 2.5826) (70.9703, 2.5023) (71.1176, 2.4211) (71.2352, 2.3556) (71.3234, 2.3061) (71.3821, 2.2729) (71.4115, 2.2563) knots 0 0 0 0 0 0 0.01428571 0.02857143 0.04285714 0.05714286 0.07142857 0.08571429 0.1 0.11428571 0.12857143 0.14285714 0.15714286 0.17142857 0.18571429 0.2 0.21428571 0.22857143 0.24285714 0.25714286 0.27142857 0.28571429 0.3 0.31428571 0.32857143 0.34285714 0.35714286 0.37142857 0.38571429 0.4 0.41428571 0.42857143 0.44285714 0.45714286 0.47142857 0.48571429 0.5 0.51428571 0.52857143 0.54285714 0.55714286 0.57142857 0.58571429 0.6 0.61428571 0.62857143 0.64285714 0.65714286 0.67142857 0.68571429 0.7 0.71428571 0.72857143 0.74285714 0.75714286 0.77142857 0.78571429 0.8 0.81428571 0.82857143 0.84285714 0.85714286 0.87142857 0.88571429 0.9 0.91428571 0.92857143 0.94285714 0.95714286 0.97142857 0.98571429 1 1 1 1 1 1
  arc A0 (71.4115, -2.2563) -> (71.4115, 2.2563) centre (0, 0) ccw
  line L0 (57.1764, -5.3584) -> (60.7685, -5.6951)
  line L1 (57.1764, 5.3584) -> (60.7685, 5.6951)
  line L2 (57.1764, -5.3584) -> (57.1764, 5.3584)
  point P0 (61.5163, -5.6869)
  point P1 (62.2698, -5.6129)
  point P2 (63.027, -5.4947)
  point P3 (63.7867, -5.3395)
  point P4 (64.5483, -5.1514)
  point P5 (65.3112, -4.9332)
  point P6 (66.075, -4.6865)
  point P7 (66.8392, -4.413)
  point P8 (67.6034, -4.1137)
  point P9 (68.3672, -3.7895)
  point P10 (69.1303, -3.4411)
  point P11 (69.8923, -3.0691)
  point P12 (70.6528, -2.674)
  point P13 (61.5163, 5.6869)
  point P14 (62.2698, 5.6129)
  point P15 (63.027, 5.4947)
  point P16 (63.7867, 5.3395)
  point P17 (64.5483, 5.1514)
  point P18 (65.3112, 4.9332)
  point P19 (66.075, 4.6865)
  point P20 (66.8392, 4.413)
  point P21 (67.6034, 4.1137)
  point P22 (68.3672, 3.7895)
  point P23 (69.1303, 3.4411)
  point P24 (69.8923, 3.0691)
  point P25 (70.6528, 2.674)
extrude "Extrude5" add sketch "Gear Tooth" along normal blind 4.2 bodies 6
fillet "Fillet2" radius 2 2 edges at (57.1864, -5.3593, 2.1) (57.1864, 5.3593, 2.1) on bodies 6
pattern_circular "C-Pattern2" count 20 over 360 about axis through (0, 0, 0) along (0, 0, 1) of "Extrude5", "Fillet2"
sketch "Diametrial Pitch Circle" plane through (0, 0, 0) normal (0, 0, 1) x (1, 0, 0)
  circle A0 centre (0, 0) radius 64.9519 construction
move_body "Move1" bodies 6 to x (0, 1, 0) y (-1, 0, 0) z (0, 0, 1) at (0, 0, 0)
sketch "Sketch10" plane through (0, 0, 0) normal (0, 0, 1) x (1, 0, 0)
  line L0 (0, 0) -> (0, 100) construction
  dimension "d70" = 100
  constraint coincident L0.start origin
  constraint vertical L0
  measures "d70" distance of L0.start L0.end